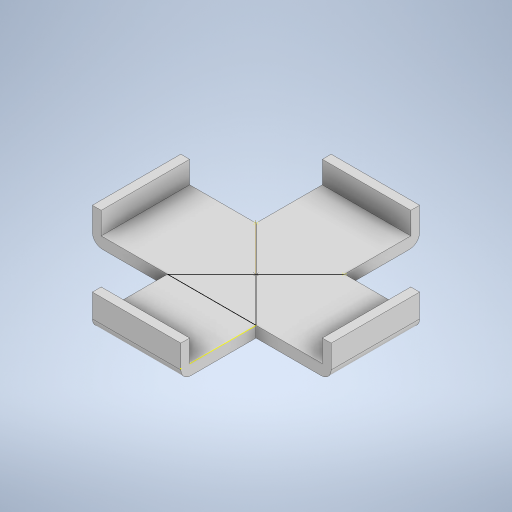
# Autodesk Inventor part: Part5
Saved by Autodesk Inventor 2023.1 (Build 271208000, 208)
## iProperties
Created: 2023-11-10
Part Number: Part5
Material: Generic
Document SubType Name: Modeling
Designer: Piotrek
Density: 1 g/cm^3
Appearance: Default
Author: Piotrek
Autodesk Inventor part; units mm, degrees
ref_plane "YZ Plane" through (0, 0, 0) normal (1, 0, 0) x (0, 1, 0)
ref_plane "XZ Plane" through (0, 0, 0) normal (0, 1, 0) x (-1, 0, 0)
ref_plane "XY Plane" through (0, 0, 0) normal (0, 0, 1) x (1, 0, 0)
sketch "Sketch1" plane through (0, 0, 0) normal (0, 1, 0) x (-1, 0, 0)
  line L0 (0, 0) -> (20, 0)
  line L1 (20, 0) -> (20, -54)
  line L2 (20, -54) -> (0, -54)
  line L3 (0, -54) -> (0, 0)
  line L4 (20, -27) -> (0, -27)
  line L5 (-17, -17) -> (37, -17)
  line L6 (37, -17) -> (37, -37)
  line L7 (37, -37) -> (-17, -37)
  line L8 (-17, -37) -> (-17, -17)
  line L9 (-17, -17) -> (37, -37) construction
  line L10 (37, -17) -> (-17, -37) construction
  point P0 (10, -27)
  point P1 (0, -17)
  point P2 (0, -37)
  point P3 (20, -37)
  point P4 (20, -17)
  dimension "d0" = 20
  dimension "d1" = 54
  dimension "d2" = 54
  dimension "d3" = 20
  constraints: 22 end point, 5 midpoint, 4 parallel, 2 horizontal, 2 perpendicular
  measures "d0" distance of L1.end L2.end
  measures "d1" distance of L0.end L1.end
  measures "d2" distance of L6.end L7.end
  measures "d3" distance of L5.end L6.end
extrude "Extrusion1" add sketch "Sketch1" along normal blind 2.5
sketch "Sketch2" plane through (0, 2.5, 0) normal (0, 1, 0) x (1, 0, 0)
  line L0 (-20, 0) -> (0, 0) projected
  line L1 (0, 0) -> (0, 17) projected
  line L2 (-20, 0) -> (0, 0)
  line L3 (0, 0) -> (0, 2)
  line L4 (0, 2) -> (-20, 2)
  line L5 (-20, 2) -> (-20, 0)
  dimension "d6" = 2
  constraints: 8 end point, 2 parallel, 1 horizontal, 1 perpendicular, 1 point on line
  measures "d6" distance of L3.end L2.end
extrude "Extrusion2" add sketch "Sketch2" along normal blind 5
sketch "Sketch3" plane through (0, 2.5, 0) normal (0, 1, 0) x (1, 0, 0)
  line L0 (0, 2) -> (0, 17) projected
  line L1 (-20, 37) -> (0, 17)
  line L2 (0, 17) -> (-20, 17)
  line L3 (-20, 17) -> (0, 37)
  point P0 (0, 0)
  point P1 (-10, 27)
  constraints: 6 end point, 2 perpendicular, 1 midpoint
pattern_circular "Circular Pattern1" count 4 over 360 about axis through (-10, 2.5, -27) along (0, 1, 0) of "Extrusion2"
fillet "Fillet1" radius 2.25 4 edges at (-10, 0, 0) (-37, 0, -27) (-10, 0, -54) (17, 0, -27)
body "Solid1"
